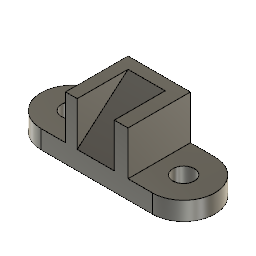
A2 (Autodesk Fusion 360 design; units mm, degrees)
Autodesk Fusion 360 part; units mm, degrees
sketch "Sketch1" plane through (0, 0, 0) normal (0, 0, 1) x (1, 0, 0)
  line L0 (57, -32) -> (-57, -32)
  line L1 (-57, 32) -> (57, 32)
  line L2 (-32, -32) -> (32, -32)
  line L3 (32, -32) -> (32, 32)
  line L4 (32, 32) -> (-32, 32)
  circle A0 centre (-57, 0) radius 11
  circle A1 centre (57, 0) radius 11
  line L5 (-32, 19.975) -> (-32, 17.9649)
  line L6 (-32, -17.9649) -> (-32, -32)
  arc A2 (-57, 32) -> (-57, -32) centre (-57, 0) ccw
  arc A3 (57, -32) -> (57, 32) centre (57, 0) ccw
  line L7 (-32, 19.975) -> (-32, -17.9649)
  line L8 (-32, 32) -> (-32, 17.9649)
  line L9 (-19.9875, 20) -> (18.0125, 20)
  line L10 (-19.9875, 20) -> (-19.9875, -32)
  line L11 (18.0125, 20) -> (18.0125, -32)
  dimension "d1" = 114
  dimension "d2" = 64
  dimension "d3" = 64
  dimension "d7" = 22
  dimension "d8" = 22
  dimension "d10" = 38
  dimension "d11" = 180
  constraint horizontal L0
  constraint parallel L0 L1
  constraint horizontal L2
  constraint vertical L3
  constraint horizontal L4
  constraint vertical L5
  constraint coincident L1 L3.end
  constraint coincident L0 L2.start
  constraint collinear L5 L6
  constraint perpendicular L1 L8
  constraint horizontal L9
  constraint coincident L0 L10.end
  constraint perpendicular L2 L11
  constraint coincident L0 L11.end
  measures "d1" distance of L1.start L1.end
  measures "d2" distance of L0.end L1.start
  measures "d3" distance of L3.end L4.end
  measures "d7" diameter of A0
  measures "d8" diameter of A1
  measures "d10" distance of L9.start L9.end
  measures "d11" angle of L10 L11
extrude "Extrude1" add sketch "Sketch1" along normal blind 19 contours L0 L1 L3 A3 | L0 L1 L5 L6 A2 L7 L8 makes body 1 at (-46.8333, 24.5088, 0) makes body 2 at (46.8333, 24.5088, 0)
extrude "Extrude2" add sketch "Sketch1" along normal blind 64 contours L0 L1 L2 L3 L4 L5 L6 L7 L8 L9 L10 L11 bodies 1 2
extrude "Extrude3" add sketch "Sketch1" along normal blind 19 contours L0 L2 L9 L10 L11 bodies 1
sketch "Sketch2" plane through (0, 0, 0) normal (1, 0, 0) x (0, 1, 0)
  line L0 (20, 64, -19.9875) -> (20, 64, 18.0125)
  line L1 (-32, 19, -19.9875) -> (-32, 19, 18.0125)
  line L2 (20, 64, -0.9875) -> (-32, 19, -0.9875)
  line L3 (20, 19, -19.9875) -> (20, 19, 18.0125)
  line L4 (20, 19, -0.9875) -> (20, 64, -0.9875)
  line L5 (-32, 19, -0.9875) -> (20, 19, -0.9875)
extrude "Extrude4" add sketch "Sketch2" along normal mid plane 38 separate body contours L2 L4 L5 in plane through (-0.9875, 0, 0) normal (1, 0, 0) makes body 3
